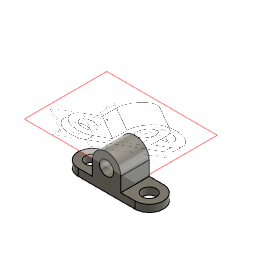
A4 v1 (Autodesk Fusion 360 design; units mm, degrees)
Autodesk Fusion 360 part; units mm, degrees
note: some values were not read from the file. Set by a fixed rule: which sketch regions a step uses.
sketch "Sketch1" plane through (0, 0, 0) normal (0, 1, 0) x (1, 0, 0)
  line L0 (40, -40) -> (80, -40)
  line L1 (80, -40) -> (80, -80)
  line L2 (80, -80) -> (40, -80)
  line L3 (40, -80) -> (40, -40)
  line L4 (80, -40) -> (100, -40)
  line L5 (100, -40) -> (100, -80)
  line L6 (100, -80) -> (80, -80)
  line L7 (40, -80) -> (20, -80)
  line L8 (20, -80) -> (20, -40)
  line L9 (20, -40) -> (40, -40)
  line L10 (20, -60) -> (100, -60)
  circle A0 centre (20, -60) radius 20
  circle A1 centre (100, -60) radius 20
  circle A2 centre (100, -60) radius 10
  circle A3 centre (20, -60) radius 10
  dimension "d1" = 40
  dimension "d2" = 40
  dimension "d3" = 20
  dimension "d4" = 40
  dimension "d5" = 40
  dimension "d6" = 20
  dimension "d7" = 20
  constraint horizontal L0
  constraint vertical L1
  constraint horizontal L2
  constraint vertical L3
  constraint perpendicular L1 L4
  constraint perpendicular L0 L5
  constraint perpendicular L1 L6
  constraint perpendicular L3 L7
  constraint perpendicular L7 L8
  constraint perpendicular L3 L9
  constraint coincident L8 L10.start
  constraint coincident L5 L10.end
  constraint perpendicular L5 L10
  constraint coincident L10.start A0.centre
  constraint coincident L10.end A1.centre
  constraint concentric A0 A3
  measures "d1" distance of L0.start L0.end
  measures "d2" distance of L0.start L2.end
  measures "d3" distance of L9 L10
  measures "d4" diameter of A0
  measures "d5" diameter of A1
  measures "d6" diameter of A2
  measures "d7" diameter of A3
extrude "Extrude1" add sketch "Sketch1" against normal blind 10 contours L0 L1 L3 L10 | L3 L9 A0 | L1 L4 A1 | L1 L2 L3 L10 | L8 L10 A0 A3 | L8 L10 A0 A3 | L3 L7 A0 | L8 A0 A3 | L1 L6 A1 | L5 L10 A1 A2 | L5 L10 A1 A2 | L5 A1 A2
extrude "Extrude2" add sketch "Sketch1" along normal blind 40 contours L0 L1 L3 L10 | L1 L2 L3 L10
fillet "Fillet1" radius 20 1 edges at (80, 40, 60)
fillet "Fillet2" radius 20 1 edges at (40, 40, 60)
sketch "Sketch2" plane through (0, 0, 40) normal (0, 0, -1) x (-1, 0, 0)
  arc A0 (-40, 20) -> (-80, 20) centre (-60, 20) ccw
  line L0 (-80, 20) -> (-80, 0)
  line L1 (-80, 0) -> (-100, 0)
  line L2 (-100, 0) -> (-100, -10)
  line L3 (-100, -10) -> (-20, -10)
  line L4 (-20, -10) -> (-20, 0)
  line L5 (-20, 0) -> (-40, 0)
  line L6 (-40, 0) -> (-40, 20)
  line L7 (-80, 0) -> (-40, 0)
  line L8 (-40, 0) -> (-40, 40)
  line L9 (-40, 40) -> (-80, 40)
  line L10 (-80, 40) -> (-80, 0)
  line L11 (-80, 40) -> (-40, 0)
  line L12 (-80, 0) -> (-40, 40)
  circle A1 centre (-60, 20) radius 10
  dimension "d16" = 40
  dimension "d17" = 40
  dimension "d18" = 20
  constraint horizontal L7
  constraint vertical L8
  constraint horizontal L9
  constraint vertical L10
  constraint coincident L0.end L1.start
  constraint coincident L5.end L6.start
  constraint concentric A0 A1
  measures "d16" distance of L8.end L9.end
  measures "d17" distance of L0.end L9.end
  measures "d18" diameter of A1
extrude "Extrude3" cut sketch "Sketch2" against normal blind 40 contours L11 L12 A1 | L11 L12 A1 | L11 L12 A1 | L11 L12 A1
named bodies: "A4"
